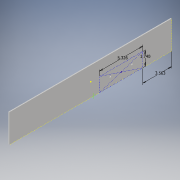
# Autodesk Inventor part: nmt_sidepanel_20in
Saved by Autodesk Inventor 2017 (Build 210142000, 142)
## iProperties
Created: 2017-02-19
Part Number: nmt_sidepanel_20in
Material: Generic
Document SubType Name: Modeling
Designer: Zara
Density: 1 g/cm^3
Appearance: Default
Author: Zara
Autodesk Inventor part; units mm, degrees
ref_plane "YZ Plane" through (0, 0, 0) normal (1, 0, 0) x (0, 1, 0)
ref_plane "XZ Plane" through (0, 0, 0) normal (0, 1, 0) x (-1, 0, 0)
ref_plane "XY Plane" through (0, 0, 0) normal (0, 0, 1) x (1, 0, 0)
sketch "Sketch1" plane through (0, 0, 0) normal (1, 0, 0) x (0, 1, 0)
  line L0 (-44.069, 254) -> (44.069, 254)
  line L1 (44.069, 254) -> (44.069, -254)
  line L2 (44.069, -254) -> (-44.069, -254)
  line L3 (-44.069, -254) -> (-44.069, 254)
  line L4 (-44.069, 254) -> (44.069, -254) construction
  line L5 (44.069, 254) -> (-44.069, -254) construction
  point P0 (0, 0)
  dimension "d0" = 508
  dimension "d1" = 88.138
  constraints: 12 end point, 2 midpoint, 2 parallel, 1 horizontal, 1 perpendicular
  measures "d0" distance of L0.end L1.end
  measures "d1" distance of L1.end L2.end
extrude "Extrusion1" add sketch "Sketch1" along normal blind 3.175
sketch "Sketch2" plane through (3.175, 0, 0) normal (1, 0, 0) x (0, 0, -1)
  line L0 (28.2321, -44.069) -> (163.5125, -44.069) construction
  line L1 (163.5125, -44.069) -> (163.5125, 0.127) construction
  line L2 (163.5125, 0.127) -> (28.2321, 0.127) construction
  line L3 (28.2321, 0.127) -> (28.2321, -44.069) construction
  line L4 (28.2321, -44.069) -> (163.5125, 0.127) construction
  line L5 (163.5125, -44.069) -> (28.2321, 0.127) construction
  line L6 (254, -44.069) -> (254, 44.069) construction
  line L7 (-254, -44.069) -> (254, -44.069) construction
  point P0 (0, 0)
  point P1 (95.8723, -21.971)
  point P2 (10.6003, -44.069)
  dimension "d4" = 135.2804
  dimension "d5" = 44.196
  dimension "d6" = 90.4875
  constraints: 12 end point, 2 midpoint, 2 parallel, 2 point on line, 1 horizontal, 1 perpendicular
  measures "d4" distance of L1.end L2.end
  measures "d5" distance of L0.end L1.end
  measures "d6" distance between parallel lines of L6 L1
sketch "Sketch3" plane through (3.175, 0, 0) normal (1, 0, 0) x (0, 0, -1)
  line L0 (62.0649, -17.78) -> (129.6797, -17.78) construction
  line L1 (-254, -44.069) -> (254, -44.069) construction
  line L2 (163.5125, -44.069) -> (163.5125, 0.127) construction
  line L3 (28.2321, 0.127) -> (28.2321, -44.069) construction
  point P0 (0, 0)
  dimension "d7" = 26.289
  dimension "d8" = 33.8328
  dimension "d9" = 33.8328
  constraints: 2 end point, 1 horizontal
  measures "d7" distance between parallel lines of L0 L1
  measures "d8" distance from line of L0.end L2
  measures "d9" distance from line of L3 L0.start
hole "Hole1" at (3.175, -17.78, -62.0649) at (3.175, -17.78, -129.6797) direction (-1, 0, 0) diameter 4.4958 end through all clearance for "Countersunk Flat Head Screw ISO 2009/7046" size "M4" standard "ISO"
body "Solid1"
